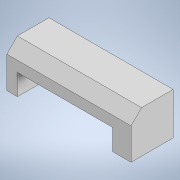
# Autodesk Inventor part: Поворотный стоппер
Saved by Autodesk Inventor 2020 (Build 240168000, 168)
## iProperties
Created: 2021-04-13
Part Number: Поворотный стоппер
Material: Типовые
Document SubType Name: Modeling
Designer: Антон
Density: 1 g/cm^3
Appearance: По умолчанию
Author: Антон
Autodesk Inventor part; units mm, degrees
ref_plane "YZ Plane" through (0, 0, 0) normal (1, 0, 0) x (0, 1, 0)
ref_plane "XZ Plane" through (0, 0, 0) normal (0, 1, 0) x (-1, 0, 0)
sketch "Эскиз1" plane through (0, 0, 0) normal (0, 0, 1) x (1, 0, 0)
  line L0 (0, 0) -> (18.1, 0)
  line L1 (18.1, 0) -> (18.1, 8)
  line L2 (18.1, 8) -> (0, 8)
  line L3 (0, 8) -> (0, 0)
  dimension "d0" = 18.1
  dimension "d1" = 8
  constraints: 8 end point, 2 parallel, 1 horizontal, 1 perpendicular
  measures "d0" distance of L2.end L1.end
  measures "d1" distance of L1.end L0.end
extrude "Выдавливание1" add sketch "Эскиз1" along normal blind 8
sketch "Эскиз2" plane through (0, 0, 8) normal (0, 0, 1) x (1, 0, 0)
  line L0 (0, 0) -> (18.1, 0) projected
  line L1 (18.1, 0) -> (18.1, 8) projected
  line L2 (0, 0) -> (18.1, 0)
  line L3 (18.1, 0) -> (18.1, 6)
  line L4 (18.1, 6) -> (0, 6)
  line L5 (0, 6) -> (0, 0)
  dimension "d4" = 6
  constraints: 8 end point, 2 parallel, 1 horizontal, 1 perpendicular, 1 point on line
  measures "d4" distance of L3.end L2.end
extrude "Выдавливание2" cut sketch "Эскиз2" against normal blind 6
ref_plane "РабПлоскость1" through (9.05, 0, 0) normal (1, 0, 0) x (0, 0, -1)
sketch "Эскиз3" plane through (18.1, 0, 0) normal (1, 0, 0) x (0, 0, -1)
  line L0 (0, 8) -> (-8, 8) projected
  line L1 (0, 8) -> (0, 0) projected
  line L2 (-8, 8) -> (0, 8)
  line L3 (0, 8) -> (0, 0)
  line L4 (0, 0) -> (-8, 0)
  line L5 (-8, 0) -> (-8, 8)
  constraints: 8 end point, 2 parallel, 1 horizontal, 1 perpendicular
extrude "Выдавливание3" add sketch "Эскиз3" along normal blind 3.5
chamfer "Фаска1" distance 2 angle 45 1 edges at (10.8, 8, 8)
sketch "Эскиз6" plane through (0, 6, 2) normal (0, -1, 0) x (1, 0, 0)
  line L0 (18.1, 6) -> (18.1, 0) projected
  line L1 (0, 6) -> (18.1, 6)
  line L2 (18.1, 6) -> (18.1, 5)
  line L3 (18.1, 5) -> (0, 5)
  line L4 (0, 5) -> (0, 6)
  line L5 (0, 0) -> (0, 6) projected
  point P0 (18, -2)
  dimension "d20" = 1
  constraints: 8 end point, 2 parallel, 1 horizontal, 1 perpendicular, 2 other
  measures "d20" distance of L1.end L2.end
extrude "Выдавливание6" add sketch "Эскиз6" along normal blind 2
sketch "Эскиз7" plane through (0, 0, 0) normal (-1, 0, 0) x (0, 0, 1)
  line L0 (8, 6) -> (6, 8) projected
  line L1 (8, 6) -> (8, 0) projected
  line L2 (8, 0) -> (0, 0) projected
  line L3 (0, 0) -> (0, 8) projected
  line L4 (0, 8) -> (6, 8) projected
extrude "Выдавливание7" add sketch "Эскиз7" along normal blind 2
